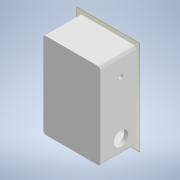
# Autodesk Inventor part: Base
Saved by Autodesk Inventor 2021 (Build 250183000, 183)
## iProperties
Created: 2020-11-13
Part Number: Base
Material: Generic
Document SubType Name: Modeling
Designer: siwat
Density: 1 g/cm^3
Appearance: Default
Author: siwat
Autodesk Inventor part; units mm, degrees
ref_plane "YZ Plane" through (0, 0, 0) normal (1, 0, 0) x (0, 1, 0)
ref_plane "XZ Plane" through (0, 0, 0) normal (0, 1, 0) x (-1, 0, 0)
ref_plane "XY Plane" through (0, 0, 0) normal (0, 0, 1) x (1, 0, 0)
ref_plane "Work Plane1" through (0, 0, 0) normal (0, 0, 1) x (1, 0, 0)
sketch "Sketch1" plane through (0, 0, 0) normal (0, 0, 1) x (1, 0, 0)
  line L0 (45, 75) -> (-45, 75)
  line L1 (-50, 70) -> (-50, -70)
  line L2 (-45, -75) -> (45, -75)
  line L3 (50, -70) -> (50, 70)
  arc A0 (50, 70) -> (45, 75) centre (45, 70) ccw
  arc A1 (-45, 75) -> (-50, 70) centre (-45, 70) ccw
  arc A2 (-50, -70) -> (-45, -75) centre (-45, -70) ccw
  arc A3 (45, -75) -> (50, -70) centre (45, -70) ccw
  line L4 (43.008, 67.9028) -> (-43.1443, 67.9028)
  line L5 (-43.1443, 67.9028) -> (-43.1443, -67.7709)
  line L6 (-43.1443, -67.7709) -> (43.008, -67.7709)
  line L7 (43.008, -67.7709) -> (43.008, 67.9028)
  circle A4 centre (45, 70) radius 1.5085
  circle A5 centre (-45, 70) radius 1.5
  circle A6 centre (-45, -70) radius 1.5
  circle A7 centre (45, -70) radius 1.5
  point P0 (0, 0)
  dimension "d0" = 5
  dimension "d1" = 3
  dimension "d2" = 3
  dimension "d3" = 3
  constraints: 16 end point, 8 centre point, 8 point on circle, 8 tangent, 4 coincident, 4 parallel, 3 equal radius, 2 horizontal, 2 perpendicular
  measures "d0" radius of A0
  measures "d1" diameter of A5
  measures "d2" diameter of A6
  measures "d3" diameter of A7
extrude "Extrusion1" add sketch "Sketch1" along normal blind 60
sketch "Sketch2" plane through (50, -70, 0) normal (1, 0, 0) x (0, 0, -1)
  circle A0 centre (-27.4102, 19.5745) radius 12.5
  circle A1 centre (-27.4102, 112.7876) radius 3.75
  point P0 (0, 70)
  dimension "d6" = 25
  dimension "d9" = 7.5
  constraints: 2 centre point
  measures "d6" diameter of A0
  measures "d9" diameter of A1
extrude "Extrusion2" cut sketch "Sketch2" against normal up to surface (6.992 mm away)
sketch "Sketch3" plane through (0, 0, 60) normal (0, 0, 1) x (1, 0, 0)
  line L0 (-45, 75) -> (45, 75)
  line L1 (50, 70) -> (50, -70)
  line L2 (45, -75) -> (-45, -75)
  line L3 (-50, -70) -> (-50, 70)
  arc A0 (45, -75) -> (50, -70) centre (45, -70) ccw
  arc A1 (-50, -70) -> (-45, -75) centre (-45, -70) ccw
  arc A2 (-45, 75) -> (-50, 70) centre (-45, 70) ccw
  arc A3 (50, 70) -> (45, 75) centre (45, 70) ccw
  point P0 (0, 0)
  dimension "d10" = 5
  constraints: 8 end point, 8 point on circle, 8 tangent, 4 centre point, 3 equal radius, 2 parallel, 1 horizontal, 1 perpendicular
  measures "d10" radius of A0
extrude "Extrusion3" add sketch "Sketch3" along normal blind 3.5625
sketch "Sketch4" plane through (-50, -70, 0) normal (-1, 0, 0) x (0, 0, 1)
  circle A0 centre (33.4987, 16.7277) radius 5.1927
  circle A1 centre (33.4987, 109.0376) radius 6.5
  point P0 (0, 70)
  dimension "d15" = 13
  constraints: 2 centre point
  measures "d15" diameter of A1
extrude "Extrusion4" cut sketch "Sketch4" against normal up to surface (6.8557 mm away)
body "Solid1"
